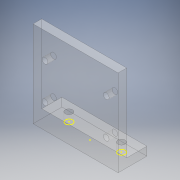
# Autodesk Inventor part: Kamera Holder
Saved by Autodesk Inventor 2017 (Build 210142000, 142)
## iProperties
Created: 2021-02-18
Part Number: Kamera Holder
Material: Generic
Document SubType Name: Modeling
Designer: Lenovo Y900
Density: 1 g/cm^3
Appearance: Polycarbonate - Clear
Author: Lenovo Y900
Autodesk Inventor part; units mm, degrees
ref_plane "YZ Plane" through (0, 0, 0) normal (1, 0, 0) x (0, 1, 0)
ref_plane "XZ Plane" through (0, 0, 0) normal (0, 1, 0) x (-1, 0, 0)
ref_plane "XY Plane" through (0, 0, 0) normal (0, 0, 1) x (1, 0, 0)
sketch "Sketch1" plane through (0, 0, 0) normal (0, 0, 1) x (1, 0, 0)
  line L0 (-12, -5) -> (12, -5)
  line L1 (12, -5) -> (12, 5)
  line L2 (12, 5) -> (-12, 5)
  line L3 (-12, 5) -> (-12, -5)
  line L4 (-12, -5) -> (12, 5) construction
  line L5 (12, -5) -> (-12, 5) construction
  line L6 (-12, 5) -> (-10, 5)
  line L7 (-12, 3) -> (-12, 5)
  line L8 (12, 5) -> (10, 5)
  line L9 (12, 3) -> (12, 5)
  circle A0 centre (-9.1253, 1.7977) radius 1.25
  circle A1 centre (9.1253, 1.7977) radius 1.25
  point P0 (0, 0)
  point P1 (-12, 0)
  point P2 (12, 0)
  point P3 (10.3753, 1.7977)
  point P4 (10.375, 1.7725)
  point P5 (9.4672, 3)
  point P6 (-9.4672, 3)
  point P7 (10.375, 1.7725)
  point P8 (-10.375, 1.7725)
  dimension "d0" = 24
  dimension "d1" = 10
  dimension "d14" = 2.5
  dimension "d15" = 2.5
  dimension "d55" = 8
  dimension "d58" = 8
  dimension "d60" = 1.625
  dimension "d61" = 1.625
  dimension "d62" = 18.2505
  constraints: 20 end point, 5 point on circle, 4 midpoint, 3 horizontal, 2 centre point, 2 parallel, 1 coincident, 1 perpendicular
  measures "d0" distance of L2.end L1.end
  measures "d1" distance of L1.end L0.end
  measures "d14" diameter of A0
  measures "d15" diameter of A1
  measures "d55" distance from line of L0 point (9.467, 3)
  measures "d58" distance from line of L0 A0.start
  measures "d60" distance from line of L1 point (10.375, 1.772)
  measures "d61" distance from line of L3 A0.end
  measures "d62" distance of A0.centre A1.centre
extrude "Extrusion4" add sketch "Sketch1" along normal blind 3
sketch "Sketch3" plane through (0, 0, 3) normal (0, 0, 1) x (1, 0, 0)
  line L0 (12, -5) -> (12, 5) projected
  line L1 (12, -5) -> (-12, -5)
  line L2 (-12, -5) -> (-12, -2)
  line L3 (-12, -2) -> (12, -2)
  line L4 (12, -2) -> (12, -5)
  point P0 (0, 0)
  point P1 (-12, -5)
  point P2 (12, 3)
  dimension "d24" = 3
  constraints: 8 end point, 2 parallel, 1 horizontal, 1 perpendicular
  measures "d24" distance of L1.end L2.end
extrude "Extrusion5" add sketch "Sketch3" along normal blind 27
sketch "Sketch4" plane through (-12, -2, 3) normal (0, 1, 0) x (1, 0, 0)
  circle A0 centre (22.625, -18.0021) radius 1
  circle A1 centre (1.375, -18.0021) radius 1
  circle A2 centre (22.625, -5.5021) radius 1
  circle A3 centre (1.375, -5.5021) radius 1
  line L0 (24, -0.0021) -> (0, -0.0021)
  line L1 (24, 0) -> (24, -27) projected
  line L2 (0, 3) -> (0, -27) projected
  point P0 (12, 3)
  dimension "d68" = 1.375
  dimension "d69" = 1.375
  dimension "d70" = 1.375
  dimension "d71" = 1.375
  constraints: 4 centre point, 2 end point, 1 horizontal
  measures "d68" distance from line of L1 A0.centre
  measures "d69" distance from line of L1 A2.centre
  measures "d70" distance from line of L2 A1.centre
  measures "d71" distance from line of L2 A3.centre
extrude "Extrusion7" cut sketch "Sketch4" against normal blind 3
sketch "Sketch5" plane through (0, 0, 0) normal (0, 0, -1) x (-1, 0, 0)
  circle A0 centre (-9.1253, 1.7977) radius 1.25 projected
  circle A1 centre (9.1253, 1.7977) radius 1.25 projected
  point P0 (0, 0)
sketch "Sketch6" plane through (-12, -5, 0) normal (-1, 0, 0) x (0, 0, 1)
  line L0 (0, 10) -> (0, 0) projected
  line L1 (0, 10) -> (3, 10) projected
  line L2 (0, 10) -> (3, 10)
  line L3 (3, 3) -> (3, 10) projected
  line L4 (3, 10) -> (3, 3)
  line L5 (30, 3) -> (30, 0) projected
  line L6 (3, 3) -> (30, 3)
  line L7 (30, 3) -> (30, 0)
  line L8 (30, 0) -> (0, 0)
  line L9 (0, 0) -> (0, 10)
  point P0 (0, 5)
  constraints: 12 end point, 4 perpendicular, 1 collinear, 1 horizontal
extrude "Extrusion8" add sketch "Sketch6" along normal blind 2.75
sketch "Sketch7" plane through (12, -5, 0) normal (1, 0, 0) x (0, 0, -1)
  line L0 (0, 0) -> (0, 10) projected
  line L1 (0, 10) -> (-3, 10) projected
  line L2 (0, 10) -> (-3, 10)
  line L3 (-3, 3) -> (-3, 10) projected
  line L4 (-3, 10) -> (-3, 3)
  line L5 (-30, 0) -> (-30, 3) projected
  line L6 (-3, 3) -> (-30, 3)
  line L7 (-30, 3) -> (-30, 0)
  line L8 (0, 0) -> (-30, 0) projected
  line L9 (-30, 0) -> (0, 0)
  line L10 (0, 0) -> (0, 10)
  point P0 (0, 5)
  constraints: 12 end point, 3 collinear, 3 perpendicular
extrude "Extrusion9" add sketch "Sketch7" along normal blind 2.75
body "Solid3"
